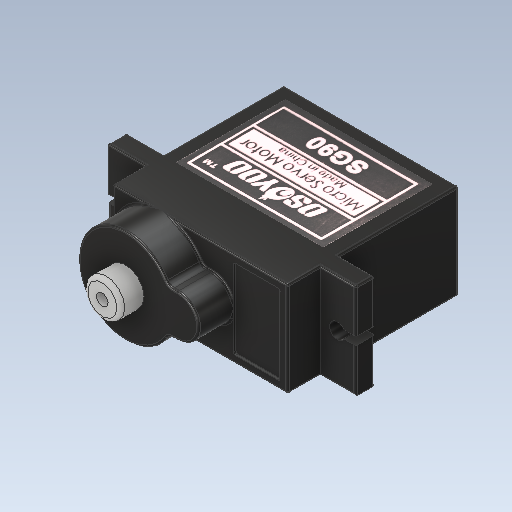
# Autodesk Inventor part: SG90
Saved by Autodesk Inventor 2020 (Build 240168000, 168)
## iProperties
Created: 2018-08-26
Part Number: SG90
Material: ABS Plastic
Document SubType Name: Modeling
Designer: henri
Density: 1.06 g/cm^3
Appearance: Smooth - White
Author: henri
Autodesk Inventor part; units mm, degrees
ref_plane "YZ Plane" through (0, 0, 0) normal (1, 0, 0) x (0, 1, 0)
ref_plane "XZ Plane" through (0, 0, 0) normal (0, 1, 0) x (-1, 0, 0)
sketch "Sketch1" plane through (0, 0, 0) normal (0, 0, 1) x (1, 0, 0)
  line L0 (0, 0) -> (22.6, 0)
  line L1 (22.6, 0) -> (22.6, 12.3)
  line L2 (22.6, 12.3) -> (0, 12.3)
  line L3 (0, 12.3) -> (0, 0)
  dimension "d0" = 22.6
  dimension "d1" = 12.3
  constraints: 8 end point, 2 parallel, 1 horizontal, 1 perpendicular
  measures "d0" distance of L2.end L1.end
  measures "d1" distance of L1.end L0.end
extrude "Extrusion1" add sketch "Sketch1" along normal blind 22.1
ref_plane "Work Plane1" through (0, 0, 15.5) normal (0, 0, 1) x (1, 0, 0)
sketch "Sketch2" plane through (0, 0, 15.5) normal (0, 0, 1) x (1, 0, 0)
  point P0 (0, 0)
sketch "Sketch3" plane through (0, 0, 15.5) normal (0, 0, 1) x (1, 0, 0)
  line L0 (-4.8, 0) -> (27.2, 0)
  line L1 (27.2, 0) -> (27.2, 12.3)
  line L2 (27.2, 12.3) -> (-4.8, 12.3)
  line L3 (-4.8, 12.3) -> (-4.8, 0)
  point P0 (0, 0)
  dimension "d5" = 32
  constraints: 8 end point, 2 parallel, 1 horizontal, 1 perpendicular
  measures "d5" distance of L2.end L1.end
extrude "Extrusion2" add sketch "Sketch3" along normal blind 2.4
sketch "Sketch4" plane through (0, 0, 17.9) normal (0, 0, 1) x (1, 0, 0)
  line L0 (0, 12.3) -> (0, 0) projected
  line L1 (-4.8, 12.3) -> (-4.8, 0) projected
  circle A0 centre (-2.4, 6.15) radius 1
  circle A1 centre (24.8, 6.15) radius 1
  line L2 (-4.8, 6.65) -> (-3.266, 6.65)
  line L3 (-3.266, 6.65) -> (-3.266, 5.65)
  line L4 (-3.266, 5.65) -> (-4.8, 5.65)
  line L5 (-4.8, 5.65) -> (-4.8, 6.65)
  line L6 (27.2, 0) -> (27.2, 12.3) projected
  line L7 (27.2, 6.65) -> (25.666, 6.65)
  line L8 (25.666, 6.65) -> (25.666, 5.65)
  line L9 (25.666, 5.65) -> (27.2, 5.65)
  line L10 (27.2, 5.65) -> (27.2, 6.65)
  point P0 (0, 6.15)
  point P1 (-4.8, 6.15)
  point P2 (27.2, 6.15)
  dimension "d8" = 2
  dimension "d9" = 2
  dimension "d10" = 1
  dimension "d11" = 1
  constraints: 16 end point, 4 parallel, 3 midpoint, 2 coincident, 2 horizontal, 2 perpendicular, 2 point on line, 6 other
  measures "d10" distance of L2.end L3.end
  measures "d11" distance of L8.end L7.end
extrude "Extrusion3" cut sketch "Sketch4" against normal blind 2.4
sketch "Sketch5" plane through (0, 0, 22.1) normal (0, 0, 1) x (1, 0, 0)
  line L0 (0, 0) -> (22.6, 0) projected
  line L1 (22.6, 0) -> (22.6, 12.3) projected
  line L2 (22.6, 12.3) -> (0, 12.3) projected
  line L3 (0, 12.3) -> (0, 0) projected
  circle A0 centre (6.15, 6.15) radius 6.15
  constraints: 3 tangent, 1 centre point
extrude "Extrusion4" add sketch "Sketch5" along normal blind 4.5 contours A0
sketch "Sketch6" plane through (0, 0, 22.1) normal (0, 0, 1) x (1, 0, 0)
  line L0 (21.6, 1) -> (15.6, 1)
  line L1 (15.6, 1) -> (15.6, 11.3)
  line L2 (15.6, 11.3) -> (21.6, 11.3)
  line L3 (21.6, 11.3) -> (21.6, 1)
  point P0 (0, 0)
  dimension "d16" = 6
  dimension "d17" = 10.3
  constraints: 8 end point, 2 parallel, 1 horizontal, 1 perpendicular
  measures "d16" distance of L1.end L2.end
  measures "d17" distance of L0.end L1.end
extrude "Extrusion5" cut sketch "Sketch6" against normal blind 0.3
sketch "Sketch7" plane through (0, 0, 22.1) normal (0, 0, 1) x (1, 0, 0)
  arc A0 (6.15, 0) -> (6.15, 12.3) centre (6.15, 6.15) ccw projected
  line L0 (15.6, 1) -> (15.6, 11.3) projected
  circle A1 centre (12.85, 6.15) radius 2.75
  line L1 (10.1, 8.9) -> (12.85, 8.9)
  line L2 (12.85, 8.9) -> (12.85, 3.4)
  line L3 (12.85, 3.4) -> (10.1, 3.4)
  line L4 (10.1, 3.4) -> (10.1, 8.9)
  point P0 (0, 0)
  point P1 (15.6, 6.15)
  constraints: 8 end point, 2 parallel, 2 point on circle, 1 centre point, 1 coincident, 1 horizontal, 1 midpoint, 1 perpendicular
extrude "Extrusion6" add sketch "Sketch7" along normal blind 4.5
fillet "Fillet1" radius 1 2 edges at (11.6509, 3.4, 24.35) (11.6509, 8.9, 24.35)
sketch "Sketch8" plane through (0, 0, 26.6) normal (0, 0, 1) x (1, 0, 0)
  arc A0 (6.15, 12.3) -> (0, 6.15) centre (6.15, 6.15) ccw projected
  circle A1 centre (6.15, 6.15) radius 2.4
  circle A2 centre (6.15, 6.15) radius 0.75
  point P0 (0, 0)
  dimension "d23" = 4.8
  dimension "d24" = 1.5
  constraints: 3 coincident, 2 centre point
  measures "d23" diameter of A1
  measures "d24" diameter of A2
extrude "Extrusion7" add sketch "Sketch8" along normal blind 3 separate body
fillet "Fillet2" radius 0.5 1 edges at (3.75, 6.15, 29.6)
fillet "Fillet3" radius 0.25 4 edges at (15.6, 11.3, 21.95) (21.6, 11.3, 21.95) (15.6, 1, 21.95) (21.6, 1, 21.95)
fillet "Fillet4" radius 0.25 1 edges at (3.075, 12.3, 22.1)
fillet "Fillet5" radius 0.25 1 edges at (14.375, 12.3, 22.1)
fillet "Fillet6" radius 0.25 1 edges at (3.075, 0, 22.1)
fillet "Fillet7" radius 0.25 1 edges at (14.375, 0, 22.1)
fillet "Fillet8" radius 0.25 3 edges at (0, 0.0732, 22.0268) (0, 0, 19.875) (0, 3.2, 22.1)
fillet "Fillet9" radius 0.25 3 edges at (0, 12.2268, 22.0268) (0, 12.3, 19.875) (0, 9.1, 22.1)
fillet "Fillet10" radius 0.25 18 edges at (11.7501, 3.2731, 26.6) (12.5438, 3.4, 26.6) (15.6, 6.15, 26.6) (12.5438, 8.9, 26.6) (11.7501, 9.0269, 26.6) (0, 6.15, 26.6) (22.6, 12.2268, 22.0268) (22.6, 12.3, 19.875) (22.6, 0.0732, 22.0268) (22.6, 0, 19.875) (22.6, 6.15, 22.1) (22.6, 0, 7.75) (22.6, 12.3, 7.75) (22.6, 6.15, 0) (11.3, 0, 0) (0, 0, 7.75) (0, 12.3, 7.75) (11.3, 12.3, 0)
fillet "Fillet11" radius 0.25 13 edges at (22.475, 0, 17.9) (24.9, 0, 17.9) (27.2, 2.825, 17.9) (27.2, 9.475, 17.9) (22.475, 12.3, 17.9) (24.9, 12.3, 17.9) (27.2, 12.3, 16.7) (27.2, 9.475, 15.5) (27.2, 2.825, 15.5) (24.9, 0, 15.5) (22.475, 0, 15.5) (24.9, 12.3, 15.5) (22.475, 12.3, 15.5)
fillet "Fillet12" radius 0.25 10 edges at (-2.275, 0, 17.9) (-4.8, 2.825, 17.9) (-4.8, 2.825, 15.5) (0.125, 0, 15.5) (-2.4, 0, 15.5) (-2.275, 12.3, 17.9) (-4.8, 9.475, 15.5) (-4.8, 12.3, 16.7) (-2.4, 12.3, 15.5) (0.125, 12.3, 15.5)
sketch "Sketch9" plane through (0, 0.25, 0) normal (-1, 0, 0) x (0, 0, 1)
  circle A0 centre (5, 5.9) radius 0.5
  point P0 (0, -0.25)
  dimension "d38" = 1
  constraints: 1 centre point, 1 coincident
  measures "d38" diameter of A0
extrude "Extrusion8" add sketch "Sketch9" along normal blind 3 separate body
sketch "Sketch10" plane through (0, 0.25, 0) normal (-1, 0, 0) x (0, 0, 1)
  circle A0 centre (5, 6.9) radius 0.5
  point P0 (0, -0.25)
  dimension "d41" = 1
  constraints: 1 centre point
  measures "d41" diameter of A0
extrude "Extrusion9" add sketch "Sketch10" along normal blind 3 separate body
sketch "Sketch11" plane through (0, 0.25, 0) normal (-1, 0, 0) x (0, 0, 1)
  circle A0 centre (5, 4.9) radius 0.5
  point P0 (0, -0.25)
  dimension "d44" = 1
  constraints: 1 centre point
  measures "d44" diameter of A0
extrude "Extrusion10" add sketch "Sketch11" along normal blind 3 separate body
fillet "Fillet13" radius 0.25 16 edges at (0.0647, 5.2606, 22.0178) (5.2606, 0.0647, 22.0178) (1.8013, 1.8013, 22.1) (7.0396, 0.0647, 22.0178) (11.7501, 3.2731, 22.1) (12.5438, 3.4, 22.1) (14.7945, 4.2055, 22.1) (9.8836, 1.263, 22.1) (5.2607, 12.2354, 22.0177) (0.0647, 7.0396, 22.0178) (1.8013, 10.4987, 22.1) (11.7501, 9.0269, 22.1) (12.5438, 8.9, 22.1) (14.7945, 8.0945, 22.1) (7.0395, 12.2353, 22.0178) (9.8836, 11.037, 22.1)
sketch "Sketch12" plane through (0.25, 0, 0.25) normal (0, -1, 0) x (1, 0, 0)
  line L0 (2.0641, 15.3163) -> (20.2085, 15.3163) construction
  line L1 (20.2085, 15.3163) -> (20.2085, 1.8186) construction
  line L2 (20.2085, 1.8186) -> (2.0641, 1.8186) construction
  line L3 (2.0641, 1.8186) -> (2.0641, 15.3163) construction
  point P0 (-0.25, -0.25)
  constraints: 2 other
decal "Decal1"
sketch "Sketch13" plane through (0.25, 12.3, 0.25) normal (0, 1, 0) x (1, 0, 0)
  line L0 (20.4891, -15.4154) -> (1.4412, -15.4154) construction
  line L1 (1.4412, -15.4154) -> (1.4412, -1.2456) construction
  line L2 (1.4412, -1.2456) -> (20.4891, -1.2456) construction
  line L3 (20.4891, -1.2456) -> (20.4891, -15.4154) construction
  point P0 (-0.25, 0.25)
  constraints: 2 other
decal "Decal2"
body "Solid1"
body "Solid2"
body "Solid3"
body "Solid4"
body "Solid5"
